Up Cover (Autodesk Fusion 360 design; units mm, degrees)
Autodesk Fusion 360 part; units mm, degrees
sketch "Sketch1" plane through (0, 0, 0) normal (0, 0, 1) x (1, 0, 0) in component "Up  Cover - Back"
  line L0 (64, 138) -> (-64, 138)
  line L1 (-64, 138) -> (-64, -138)
  line L2 (-64, -138) -> (64, -138)
  line L3 (64, -138) -> (64, 138)
  line L4 (64, 138) -> (-64, -138) construction
  line L5 (-64, 138) -> (64, -138) construction
  line L6 (-64, 138) -> (-74, 138)
  line L7 (-74, 138) -> (-74, -138)
  line L8 (-74, -138) -> (-64, -138)
  line L9 (-64, -138) -> (-64, 138)
  line L10 (64, 138) -> (87.5, 138)
  line L11 (87.5, 138) -> (87.5, -138)
  line L12 (87.5, -138) -> (64, -138)
  line L13 (64, -138) -> (64, 138)
  circle A0 centre (-74, 0) radius 15
  line L14 (14, 138) -> (64, 88)
  line L15 (64, -88) -> (14, -138)
  line L16 (-74, -138) -> (87.5, -138)
  line L17 (87.5, -138) -> (87.5, -162)
  line L18 (87.5, -162) -> (-74, -162)
  line L19 (-74, -162) -> (-74, -138)
  line L20 (-74, 138) -> (87.5, 138)
  line L21 (87.5, 138) -> (87.5, 162)
  line L22 (87.5, 162) -> (-74, 162)
  line L23 (-74, 162) -> (-74, 138)
  dimension "d3" = 10
  dimension "d4" = 23.5
  dimension "d5" = 30
  dimension "d6" = 50
  dimension "d7" = 50
  dimension "d8" = 50
  dimension "d9" = 50
  dimension "d14" = 161.5
  dimension "d15" = 24
  dimension "d16" = 24
  dimension "d17" = 324
  constraint horizontal L0
  constraint perpendicular L0 L1
  constraint parallel L0 L2
  constraint parallel L1 L3
  constraint coincident L4 origin
  constraint coincident L5 origin
  constraint horizontal L6
  constraint vertical L7
  constraint horizontal L8
  constraint vertical L9
  constraint coincident L1.end L2.start
  constraint horizontal L10
  constraint vertical L11
  constraint horizontal L12
  constraint vertical L13
  constraint coincident L2.end L3.start
  constraint midpoint L7 A0.centre
  constraint coincident L0 L14.start
  constraint coincident L3 L14.end
  constraint coincident L3 L15.start
  constraint coincident L2 L15.end
  constraint horizontal L16
  constraint vertical L17
  constraint horizontal L18
  constraint vertical L19
  constraint coincident L11.end L12.start
  constraint horizontal L20
  constraint vertical L21
  constraint horizontal L22
  constraint vertical L23
  constraint coincident L10.end L11.start
  measures "d3" distance of L0.end L6.end
  measures "d4" distance of L0.start L10.end
  measures "d5" diameter of A0
  measures "d6" distance of L2.end L15.end
  measures "d7" distance of L2.end L15.start
  measures "d8" distance of L0.start L14.end
  measures "d9" distance of L0.start L14.start
  measures "d14" distance of L6.end L10.end
  measures "d15" distance of L11.end L17.end
  measures "d16" distance of L10.end L21.end
  measures "d17" distance of L18.end L22.end
extrude "Extrude1" add sketch "Sketch1" against normal blind 3 contours L0 L3 L13 L14 L20 | L3 L10 L11 L12 L13 L16 L20 | L0 L6 L10 L20 L21 L22 L23 | L0 L1 L2 L3 L9 L13 A0 L14 L15 L16 L20 | L1 L6 L7 L9 A0 L20 | L2 L3 L13 L15 L16 | L2 L8 L12 L16 L17 L18 L19 | L1 L7 L8 L9 A0 L16 makes body 1 in component "Up  Cover - Back"
extrude "Extrude2" add sketch "Sketch1" along normal blind 5 contours L0 L1 L2 L3 L9 L13 A0 L14 L15 L16 L20 bodies 1 in component "Up  Cover - Back"
sketch "Sketch2" plane through (0, 0, 5) normal (0, 0, 1) x (-1, 0, 0) in component "Up  Cover - Back"
  line L0 (-14, -138) -> (64, -138)
  line L1 (64, -138) -> (64, -11.1803)
  arc A0 (64, 11.1803) -> (64, -11.1803) centre (74, 0) ccw
  line L2 (64, 11.1803) -> (64, 138)
  line L3 (64, 138) -> (-14, 138)
  line L4 (-14, 138) -> (-64, 88)
  line L5 (-64, 88) -> (-64, -88)
  line L6 (-64, -88) -> (-14, -138)
  line L7 (59.8579, -5) -> (-64, -5)
  line L8 (59.8579, 5) -> (-64, 5)
  line L9 (-64, -5) -> (-60, -5)
  line L10 (-60, -5) -> (-60, -25)
  line L11 (-60, -25) -> (-64, -25)
  line L12 (-64, -25) -> (-64, -5)
  line L13 (59.8579, -5) -> (55.8579, -5)
  line L14 (55.8579, -5) -> (55.8579, -25)
  line L15 (55.8579, -25) -> (59.8579, -25)
  line L16 (59.8579, -25) -> (59.8579, -5)
  line L17 (55.8579, -15) -> (-60, -15) construction
  line L18 (-4.0711, -5) -> (-0.0711, -5)
  line L19 (-0.0711, -5) -> (-0.0711, -25)
  line L20 (-0.0711, -25) -> (-4.0711, -25)
  line L21 (-4.0711, -25) -> (-4.0711, -5)
  line L22 (-4.0711, -5) -> (-0.0711, -25) construction
  line L23 (-0.0711, -5) -> (-4.0711, -25) construction
  line L24 (59, 0) -> (-64, 0) construction
  line L25 (59.8579, 5) -> (55.8579, 5)
  line L26 (55.8579, 25) -> (59.8579, 25)
  line L27 (59.8579, 25) -> (59.8579, 5)
  line L28 (55.8579, 5) -> (55.8579, 25)
  line L29 (-0.0711, 5) -> (-0.0711, 25)
  line L30 (-0.0711, 25) -> (-4.0711, 25)
  line L31 (-4.0711, 5) -> (-0.0711, 5)
  line L32 (-4.0711, 25) -> (-4.0711, 5)
  line L33 (-64, 5) -> (-60, 5)
  line L34 (-60, 25) -> (-64, 25)
  line L35 (-64, 25) -> (-64, 5)
  line L36 (-60, 5) -> (-60, 25)
  point P0 (-2.0711, -15)
  dimension "d18" = 5
  dimension "d19" = 5
  dimension "d20" = 20
  dimension "d21" = 4
  dimension "d22" = 4
  dimension "d23" = 20
  dimension "d24" = 4
  dimension "d25" = 20
  constraint coincident A0 L7.start
  constraint coincident L5 L7.end
  constraint perpendicular L5 L7
  constraint coincident A0 L8.start
  constraint coincident L5 L8.end
  constraint perpendicular L5 L8
  constraint horizontal L9
  constraint vertical L10
  constraint horizontal L11
  constraint vertical L12
  constraint horizontal L13
  constraint vertical L14
  constraint horizontal L15
  constraint vertical L16
  constraint midpoint L14 L17.start
  constraint midpoint L10 L17.end
  constraint horizontal L18
  constraint perpendicular L18 L19
  constraint parallel L18 L20
  constraint parallel L19 L21
  constraint coincident L22 P0
  constraint coincident L23 P0
  constraint midpoint L17 P0
  constraint midpoint A0 L24.start
  constraint midpoint L5 L24.end
  constraint symmetric L7.start L24 L8.start
  constraint symmetric L7.end L24 L8.end
  constraint symmetric L9.end L24 L33.end
  constraint symmetric L10.end L24 L34.start
  constraint symmetric L11.end L24 L34.end
  constraint symmetric L13.end L24 L25.end
  constraint symmetric L14.end L24 L26.start
  constraint symmetric L15.end L24 L26.end
  constraint symmetric L18.start L24 L31.start
  constraint symmetric L18.end L24 L29.start
  constraint symmetric L19.end L24 L29.end
  constraint symmetric L20.end L24 L30.end
  measures "d18" vertical distance of origin L8.end
  measures "d19" vertical distance of origin L7.end
  measures "d20" distance of L7.end L11.end
  measures "d21" distance of L10.end L11.end
  measures "d22" distance of L7.start L13.end
  measures "d23" distance of L7.start L15.end
  measures "d24" distance of L19.end L20.end
  measures "d25" distance of L18.end L19.end
extrude "Extrude3" add sketch "Sketch2" along normal blind 20 contours L5 L7 L9 L10 L11 L12 | A0 L5 L7 L8 L9 L13 L18 L25 L31 L33 | L7 L13 L14 L15 L16 | L8 L25 L26 L27 L28 | L5 L8 L33 L34 L35 L36 | L7 L18 L19 L20 L21 | L8 L29 L30 L31 L32 bodies 1 in component "Up  Cover - Back"
chamfer "Chamfer1" distance 20 angle 45 6 edges at (-57.8579, -25, 25) (-57.8579, 25, 25) (2.0711, -25, 25) (2.0711, 25, 25) (62, 25, 25) (62, -25, 25) on bodies 1 in component "Up  Cover - Back"
sketch "Sketch3" plane through (0, -5, 0) normal (0, -1, 0) x (1, 0, 0) in component "Up  Cover - Back"
  line L0 (-55.8579, 5) -> (0.0711, 5)
  line L1 (0.0711, 5) -> (0.0711, 25)
  line L2 (0.0711, 25) -> (-55.8579, 25)
  line L3 (-55.8579, 25) -> (-55.8579, 5)
  line L4 (4.0711, 5) -> (60, 5)
  line L5 (60, 5) -> (60, 25)
  line L6 (60, 25) -> (4.0711, 25)
  line L7 (4.0711, 25) -> (4.0711, 5)
  line L8 (-55.8579, 15) -> (60, 15) construction
  circle A0 centre (-49.8579, 15) radius 2.1
  circle A1 centre (-15.8579, 15) radius 2.1
  circle A2 centre (20, 15) radius 2.1
  line L9 (32.0355, 25) -> (32.0355, 5) construction
  line L10 (-27.8934, 25) -> (-27.8934, 5) construction
  circle A3 centre (54, 15) radius 2.1
  line L11 (-59.8579, 25) -> (-59.8579, 5)
  line L12 (64, 5) -> (64, 25)
  dimension "d29" = 4.2
  dimension "d30" = 4.2
  dimension "d31" = 4.2
  dimension "d32" = 4.2
  dimension "d33" = 10
  dimension "d34" = 10
  dimension "d35" = 34
  dimension "d36" = 34
  constraint midpoint L3 L8.start
  constraint midpoint L5 L8.end
  constraint coincident L8 A0.centre
  constraint coincident L8 A1.centre
  constraint coincident L8 A2.centre
  constraint midpoint L6 L9.start
  constraint midpoint L4 L9.end
  constraint midpoint L2 L10.start
  constraint midpoint L0 L10.end
  constraint coincident L8 A3.centre
  measures "d29" diameter of A0
  measures "d30" diameter of A1
  measures "d32" diameter of A3
  measures "d33" distance of A0.centre L11
  measures "d34" distance of A3.centre L12
  measures "d35" distance of A0.centre A1.centre
  measures "d36" distance of A2.centre A3.centre
extrude "Extrude4" cut sketch "Sketch3" against normal through all contours A0 | A1 | A2 | A3 bodies 1 in component "Up  Cover - Back"
split "Split1" by plane through (0, 0, 0) normal (0, 1, 0) bodies 1 makes body 2 at (-16.8924, 111.7787, -3) in component "Up  Cover - Back"
component "Up  Cover - Back" placed x (1, 0, 0) y (0, 1, 0) z (0, 0, 1) at (0, 0, 0)
named bodies: "Up  Cover - Back Right", "Up  Cover - Back Left"
